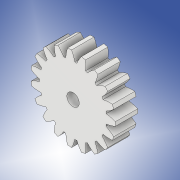
# Autodesk Inventor part: BA009
Saved by Autodesk Inventor 2017 SP1 (Build 210196100, 196)
## iProperties
Created: 2017-06-16
Part Number: BA009
Material: ABS Plastic
Document SubType Name: Modeling
Designer: Zach
Density: 1.06 g/cm^3
Appearance: CR White
Author: Zach
Autodesk Inventor part; units mm, degrees
ref_plane "YZ Plane" through (0, 0, 0) normal (1, 0, 0) x (0, 1, 0)
ref_plane "XZ Plane" through (0, 0, 0) normal (0, 1, 0) x (-1, 0, 0)
ref_plane "XY Plane" through (0, 0, 0) normal (0, 0, 1) x (1, 0, 0)
sketch "Sketch1" plane through (0, 0, 0) normal (0, 0, 1) x (1, 0, 0)
  circle A0 centre (0, 0) radius 7.5
  circle A1 centre (0, 0) radius 2.75
  dimension "d0" = 15
  dimension "d1" = 5.5
  constraints: 2 centre point, 2 coincident
  measures "d0" diameter of A0
  measures "d1" diameter of A1
extrude "Extrusion1" add sketch "Sketch1" along normal blind 5
sketch "Sketch2" plane through (0, 0, 5) normal (0, 0, 1) x (1, 0, 0)
  circle A0 centre (0, 0) radius 15
  arc A1 (18.8661, 0.9) -> (14.8661, 2) centre (12.9269, -12.8741) ccw
  arc A2 (18.8661, -0.9) -> (18.8661, 0.9) centre (-1.1137, 0) ccw
  line L0 (0, 0) -> (23.4972, 0) construction
  arc A3 (14.8661, -2) -> (18.8661, -0.9) centre (12.9269, 12.8741) ccw
  arc A4 (14.8661, -2) -> (14.8661, 2) centre (0, 0) ccw
  arc A5 (17.5516, 6.977) -> (13.4112, 6.7186) centre (16.4067, -7.9792) ccw
  arc A6 (18.1361, 5.2746) -> (17.5516, 6.977) centre (-1.0533, -0.3616) ccw
  arc A7 (14.71, 2.9354) -> (18.1361, 5.2746) centre (8.0463, 16.3739) ccw
  arc A8 (14.71, 2.9354) -> (13.4112, 6.7186) centre (0, 0) ccw
  arc A9 (14.3352, 12.298) -> (10.503, 10.7092) centre (18.1086, -2.2196) ccw
  arc A10 (15.4408, 10.8776) -> (14.3352, 12.298) centre (-0.8788, -0.684) ccw
  arc A11 (12.9598, 7.5526) -> (15.4408, 10.8776) centre (2.2937, 18.0994) ccw
  arc A12 (12.9598, 7.5526) -> (10.503, 10.7092) centre (0, 0) ccw
  arc A13 (9.5653, 16.2863) -> (6.4566, 13.5393) centre (17.8482, 3.7805) ccw
  arc A14 (11.0722, 15.3018) -> (9.5653, 16.2863) centre (-0.6091, -0.9323) ccw
  arc A15 (9.8053, 11.3515) -> (11.0722, 15.3018) centre (-3.7074, 17.8635) ccw
  arc A16 (9.8053, 11.3515) -> (6.4566, 13.5393) centre (0, 0) ccw
  arc A17 (3.7589, 18.5097) -> (1.7106, 14.9021) centre (15.6536, 9.371) ccw
  arc A18 (5.5038, 18.0678) -> (3.7589, 18.5097) centre (-0.2734, -1.0796) ccw
  arc A19 (5.5882, 13.9202) -> (5.5038, 18.0678) centre (-9.3068, 15.6918) ccw
  arc A20 (5.5882, 13.9202) -> (1.7106, 14.9021) centre (0, 0) ccw
  arc A21 (-2.4549, 18.7273) -> (-3.2208, 14.6501) centre (11.7627, 13.9459) ccw
  arc A22 (-0.661, 18.876) -> (-2.4549, 18.7273) centre (0.092, -1.1099) ccw
  arc A23 (0.7655, 14.9805) -> (-0.661, 18.876) centre (-13.8977, 11.8196) ccw
  arc A24 (0.7655, 14.9805) -> (-3.2208, 14.6501) centre (0, 0) ccw
  arc A25 (-8.4026, 16.9155) -> (-7.8032, 12.8106) centre (6.5971, 17.0096) ccw
  arc A26 (-6.7542, 17.6386) -> (-8.4026, 16.9155) centre (0.4474, -1.0199) ccw
  arc A27 (-4.1401, 14.4173) -> (-6.7542, 17.6386) centre (-16.9825, 6.6667) ccw
  arc A28 (-4.1401, 14.4173) -> (-7.8032, 12.8106) centre (0, 0) ccw
  arc A29 (-13.4398, 13.2707) -> (-11.54, 9.5828) centre (0.7166, 18.2301) ccw
  arc A30 (-12.1155, 14.4898) -> (-13.4398, 13.2707) centre (0.7543, -0.8194) ccw
  arc A31 (-8.5971, 12.2919) -> (-12.1155, 14.4898) centre (-18.227, 0.7912) ccw
  arc A32 (-8.5971, 12.2919) -> (-11.54, 9.5828) centre (0, 0) ccw
  arc A33 (-17.0206, 8.1877) -> (-14.0262, 5.3165) centre (-5.2415, 17.475) ccw
  arc A34 (-16.1639, 9.7708) -> (-17.0206, 8.1877) centre (0.9794, -0.53) ccw
  arc A35 (-12.1224, 8.8344) -> (-16.1639, 9.7708) centre (-17.4963, -5.1699) ccw
  arc A36 (-12.1224, 8.8344) -> (-14.0262, 5.3165) centre (0, 0) ccw
  arc A37 (-18.7569, 2.2175) -> (-14.9925, 0.4742) centre (-10.6316, 14.8262) ccw
  arc A38 (-18.4606, 3.993) -> (-18.7569, 2.2175) centre (1.0985, -0.1833) ccw
  arc A39 (-14.3341, 4.4196) -> (-18.4606, 3.993) centre (-14.8696, -10.5708) ccw
  arc A40 (-14.3341, 4.4196) -> (-14.9925, 0.4742) centre (0, 0) ccw
  arc A41 (-18.4606, -3.993) -> (-14.3341, -4.4196) centre (-14.8696, 10.5708) ccw
  arc A42 (-18.7569, -2.2175) -> (-18.4606, -3.993) centre (1.0985, 0.1833) ccw
  arc A43 (-14.9925, -0.4742) -> (-18.7569, -2.2175) centre (-10.6316, -14.8262) ccw
  arc A44 (-14.9925, -0.4742) -> (-14.3341, -4.4196) centre (0, 0) ccw
  arc A45 (-16.1639, -9.7708) -> (-12.1224, -8.8344) centre (-17.4963, 5.1699) ccw
  arc A46 (-17.0206, -8.1877) -> (-16.1639, -9.7708) centre (0.9794, 0.53) ccw
  arc A47 (-14.0262, -5.3165) -> (-17.0206, -8.1877) centre (-5.2415, -17.475) ccw
  arc A48 (-14.0262, -5.3165) -> (-12.1224, -8.8344) centre (0, 0) ccw
  arc A49 (-12.1155, -14.4898) -> (-8.5971, -12.2919) centre (-18.227, -0.7912) ccw
  arc A50 (-13.4398, -13.2707) -> (-12.1155, -14.4898) centre (0.7543, 0.8194) ccw
  arc A51 (-11.54, -9.5828) -> (-13.4398, -13.2707) centre (0.7166, -18.2301) ccw
  arc A52 (-11.54, -9.5828) -> (-8.5971, -12.2919) centre (0, 0) ccw
  arc A53 (-6.7542, -17.6386) -> (-4.1401, -14.4173) centre (-16.9825, -6.6667) ccw
  arc A54 (-8.4026, -16.9155) -> (-6.7542, -17.6386) centre (0.4474, 1.0199) ccw
  arc A55 (-7.8032, -12.8106) -> (-8.4026, -16.9155) centre (6.5971, -17.0096) ccw
  arc A56 (-7.8032, -12.8106) -> (-4.1401, -14.4173) centre (0, 0) ccw
  arc A57 (-0.661, -18.876) -> (0.7655, -14.9805) centre (-13.8977, -11.8196) ccw
  arc A58 (-2.4549, -18.7273) -> (-0.661, -18.876) centre (0.092, 1.1099) ccw
  arc A59 (-3.2208, -14.6501) -> (-2.4549, -18.7273) centre (11.7627, -13.9459) ccw
  arc A60 (-3.2208, -14.6501) -> (0.7655, -14.9805) centre (0, 0) ccw
  arc A61 (5.5038, -18.0678) -> (5.5882, -13.9202) centre (-9.3068, -15.6918) ccw
  arc A62 (3.7589, -18.5097) -> (5.5038, -18.0678) centre (-0.2734, 1.0796) ccw
  arc A63 (1.7106, -14.9021) -> (3.7589, -18.5097) centre (15.6536, -9.371) ccw
  arc A64 (1.7106, -14.9021) -> (5.5882, -13.9202) centre (0, 0) ccw
  arc A65 (11.0722, -15.3018) -> (9.8053, -11.3515) centre (-3.7074, -17.8635) ccw
  arc A66 (9.5653, -16.2863) -> (11.0722, -15.3018) centre (-0.6091, 0.9323) ccw
  arc A67 (6.4566, -13.5393) -> (9.5653, -16.2863) centre (17.8482, -3.7805) ccw
  arc A68 (6.4566, -13.5393) -> (9.8053, -11.3515) centre (0, 0) ccw
  arc A69 (15.4408, -10.8776) -> (12.9598, -7.5526) centre (2.2937, -18.0994) ccw
  arc A70 (14.3352, -12.298) -> (15.4408, -10.8776) centre (-0.8788, 0.684) ccw
  arc A71 (10.503, -10.7092) -> (14.3352, -12.298) centre (18.1086, 2.2196) ccw
  arc A72 (10.503, -10.7092) -> (12.9598, -7.5526) centre (0, 0) ccw
  arc A73 (18.1361, -5.2746) -> (14.71, -2.9354) centre (8.0463, -16.3739) ccw
  arc A74 (17.5516, -6.977) -> (18.1361, -5.2746) centre (-1.0533, 0.3616) ccw
  arc A75 (13.4112, -6.7186) -> (17.5516, -6.977) centre (16.4067, 7.9792) ccw
  arc A76 (13.4112, -6.7186) -> (14.71, -2.9354) centre (0, 0) ccw
  circle A77 centre (0, 0) radius 2.75
  point P0 (18.8863, 0)
  point P1 (17.863, 6.1324)
  point P2 (14.904, 11.6002)
  point P3 (10.3298, 15.811)
  point P4 (4.6363, 18.3084)
  point P5 (-1.5596, 18.8218)
  point P6 (-7.5866, 17.2956)
  point P7 (-12.7914, 13.8951)
  point P8 (-16.61, 8.9889)
  point P9 (-18.6287, 3.1086)
  point P10 (-18.6287, -3.1086)
  point P11 (-16.61, -8.9889)
  point P12 (-12.7914, -13.8951)
  point P13 (-7.5866, -17.2956)
  point P14 (-1.5596, -18.8218)
  point P15 (4.6363, -18.3084)
  point P16 (10.3298, -15.811)
  point P17 (14.904, -11.6002)
  point P18 (17.863, -6.1324)
  dimension "d4" = 30
  dimension "d5" = 15
  dimension "d6" = 4
  dimension "d7" = 1.8
  dimension "d8" = 20
  dimension "d10" = 2
  dimension "d11" = 15
  dimension "d12" = 4
  dimension "d13" = 2
  dimension "d16" = 360
  constraints: 155 point on circle, 78 centre point, 2 coincident, 2 end point, 1 concentric, 1 horizontal, 1 point on line, 248 other
  measures "d4" diameter of A0
  measures "d5" radius of A1
  measures "d6" horizontal distance of A0.start A1.start
  measures "d7" distance of A1.start A2.start
  measures "d8" radius of A2
  measures "d10" vertical distance of point (0, 0) A0.start
  measures "d11" radius of A3
  measures "d12" horizontal distance of A0.end A2.start
  measures "d13" distance from line of L0 A0.end
extrude "Extrusion2" add sketch "Sketch2" along normal blind 10 contours A0 | A0 A1 A2 A3 | A0 A5 A6 A7 | A73 A74 A75 A0 | A0 A9 A10 A11 | A69 A70 A71 A0 | A0 A13 A14 A15 | A65 A66 A67 A0 | A0 A17 A18 A19 | A61 A62 A63 A0 | A0 A21 A22 A23 | A57 A58 A59 A0 | A0 A25 A26 A27 | A53 A54 A55 A0 | A0 A29 A30 A31 | A49 A50 A51 A0 | A0 A33 A34 A35 | A45 A46 A47 A0 | A0 A37 A38 A39 | A41 A42 A43 A0 | A77
sketch "Sketch3" plane through (0, 0, 15) normal (0, 0, 1) x (1, 0, 0)
  circle A0 centre (0, 0) radius 2.75
  dimension "d22" = 5.5
  constraints: 1 centre point, 1 coincident
  measures "d22" diameter of A0
extrude "Extrusion3" cut sketch "Sketch3" against normal through all
body "Solid1"
